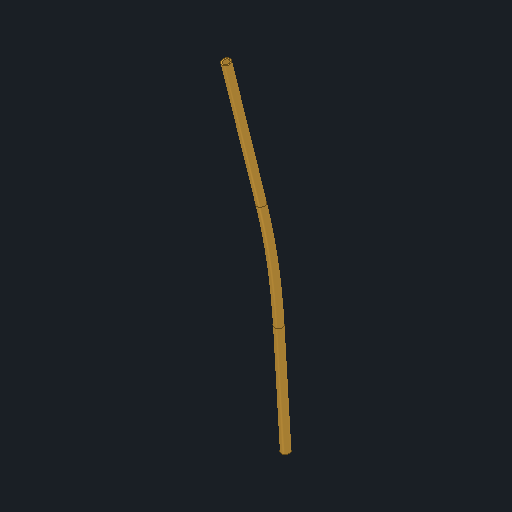
# Autodesk Inventor part: prop_shaft
Saved by Autodesk Inventor 2023 (Build 270158030, 158C)
## iProperties
Created: 2022-04-18
Part Number: prop_shaft
Material: Generic
Document SubType Name: Modeling
Designer: kardo
Density: 1 g/cm^3
Appearance: Brass - Prop shaft
Author: kardo
Autodesk Inventor part; units mm, degrees
ref_plane "YZ Plane" through (0, 0, 0) normal (1, 0, 0) x (0, 1, 0)
ref_plane "XZ Plane" through (0, 0, 0) normal (0, 1, 0) x (-1, 0, 0)
ref_plane "XY Plane" through (0, 0, 0) normal (0, 0, 1) x (1, 0, 0)
derived "stencil_frame.ipt"
sketch "sk_drivetrain_profile" plane through (6, 0, 0) normal (1, 0, 0) x (0, 1, 0)
  line L0 (-529.1913, 0) -> (410.1479, 0) construction
  line L1 (-345, 3089.1136) -> (-345, -1866.0023) construction
  line L2 (0, 3089.1136) -> (0, -1866.0023) construction
  line L3 (-134.0777, 53.4546) -> (-127.3039, 26.2863)
  line L4 (-377, 0) -> (-313.1194, 3.9071)
  line L5 (-130.6908, 39.8704) -> (-224.6958, 16.4323)
  line L6 (-301.4275, 4.6222) -> (-262.5191, 7.002) construction
  line L7 (-262.5191, 7.002) -> (-224.6958, 16.4323) construction
  line L8 (-127.3039, 26.2863) -> (-127.3039, 21.2863) construction
  line L9 (-313.1194, 3.9071) -> (-301.4275, 4.6222)
  line L10 (-869.78, 3004.1953) -> (348.339, -1881.413) construction
  line L11 (-225.3679, 19.1279) -> (-131.3629, 42.566) construction
  line L12 (-130.0187, 37.1748) -> (-224.0238, 13.7367) construction
  line L13 (-225.3679, 19.1279) -> (-224.0238, 13.7367) construction
  spline S0 degree 2 poles (-301.4275, 4.6222) (-262.5191, 7.002) (-224.6958, 16.4323) knots 1 1 1 2 2 2
  line L14 (0, 21.3303) -> (-241.5001, 18.9703) construction
  line L15 (-49.1478, 22.05) -> (-303.2844, 19.5666) construction
  point P0 (0, 0)
  point P1 (-213.4159, 19.2447)
  point P2 (-201.4639, 19.3615)
  point P3 (-196.4544, 20.6106)
ref_plane "plane_motor_mount" through (0, -120.75, 0) normal (0, 0.9702957, 0.2419219) x (-1, 0, 0)
sketch "sk_prop_shaft_profile" plane through (0, -120.75, 0) normal (0, 0.9702957, 0.2419219) x (-1, 0, 0)
  circle A0 centre (-6, 41.091) radius 2.7781
  point P0 (0, -29.2121)
  dimension "d1" = 5.5563
  constraints: 1 centre point, 1 coincident
  measures "d1" diameter of A0
derived "parameters_powertrain.ipt"
sweep "Sweep1" add profiles "sk_prop_shaft_profile" path "sk_drivetrain_profile" path curves L5 S0 L9 L4
shell "Shell1" thickness 0.7937 removed faces 2 at (5.4656, -376.9711, -0.4725) at (6.6932, -130.8394, 40.4663)
equation "\"d1\" = prop_shaft_sleeve_od"
equation "\"prop_shaft_sleeve_od\" = 5.55625"
body "Solid1"
